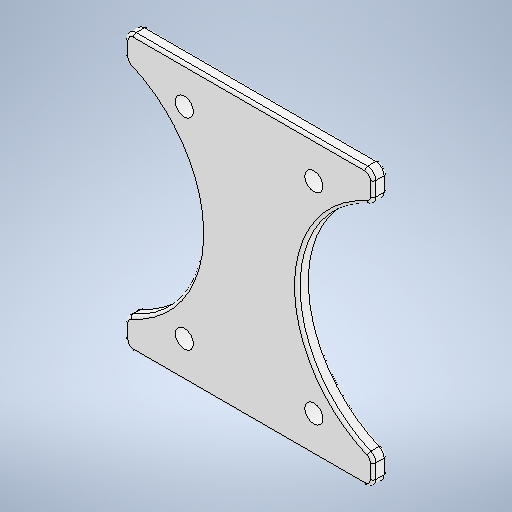
# Autodesk Inventor part: motor_clamp1
Saved by Autodesk Inventor 2025.3 (Build 293356030, 356C)
## iProperties
Created: 2025-11-17
Part Number: motor_clamp1
Material: PLA filament
Document SubType Name: Modeling
Designer: MSI
Mass: 47.447 g
Surface Area: 145.046 cm^2
Volume: 39.5392 cm^3
Density: 1.2 g/cm^3
Appearance: 일반
Author: MSI
Autodesk Inventor part; units mm, degrees
ref_plane "YZ Plane" through (0, 0, 0) normal (1, 0, 0) x (0, 1, 0)
ref_plane "XZ Plane" through (0, 0, 0) normal (0, 1, 0) x (-1, 0, 0)
ref_plane "XY Plane" through (0, 0, 0) normal (0, 0, 1) x (1, 0, 0)
sketch "스케치1" plane through (0, 0, 0) normal (0, 0, 1) x (1, 0, 0)
  line L0 (-45, 50) -> (45, 50)
  line L1 (45, 50) -> (45, -50)
  line L2 (45, -50) -> (-45, -50)
  line L3 (-45, -50) -> (-45, 50)
  line L4 (-45, 50) -> (45, -50) construction
  line L5 (45, 50) -> (-45, -50) construction
  point P0 (0, 0)
  dimension "d0" = 90
  dimension "d1" = 100
  constraints: 12 end point, 2 midpoint, 2 parallel, 1 horizontal, 1 perpendicular
  measures "d0" distance of L1.end L2.end
  measures "d1" distance of L0.end L1.end
extrude "돌출1" add sketch "스케치1" along normal mid plane 5
sketch "스케치2" plane through (0, 0, 2.5) normal (0, 0, 1) x (1, 0, 0)
  circle A0 centre (-60, 0) radius 42.5
  circle A1 centre (60, 0) radius 42.5
  point P0 (0, 0)
  dimension "d4" = 85
  dimension "d5" = 85
  dimension "d6" = 120
  dimension "d7" = 60
  constraints: 2 centre point, 2 horizontal alignment
  measures "d4" diameter of A0
  measures "d5" diameter of A1
  measures "d6" distance of A1.centre A0.centre
  measures "d7" distance of point (0, 0) A0.centre
extrude "돌출2" cut sketch "스케치2" against normal through all
sketch "스케치3" plane through (0, 0, 2.5) normal (0, 0, 1) x (1, 0, 0)
  line L0 (-23.5, 36.5) -> (23.5, 36.5) construction
  line L1 (23.5, 36.5) -> (23.5, -36.5) construction
  line L2 (23.5, -36.5) -> (-23.5, -36.5) construction
  line L3 (-23.5, -36.5) -> (-23.5, 36.5) construction
  line L4 (-23.5, 36.5) -> (23.5, -36.5) construction
  line L5 (23.5, 36.5) -> (-23.5, -36.5) construction
  point P0 (0, 0)
  dimension "d11" = 73
  dimension "d12" = 47
  constraints: 12 end point, 4 coincident, 2 midpoint, 2 parallel, 1 horizontal, 1 perpendicular
  measures "d11" distance of L0.end L1.end
  measures "d12" distance of L1.end L2.end
hole "구멍1" at (-23.5, 36.5, 2.5) at (23.5, 36.5, 2.5) at (23.5, -36.5, 2.5) at (-23.5, -36.5, 2.5) direction (0, 0, -1) diameter 6.6 end through all clearance for "Socket Head Cap Screw ISO 4762" size "M6" standard "ISO"
fillet "모깎기1" radius 3 8 edges at (45, -50, 0) (45, 50, 0) (45, 39.7649, 0) (-45, -50, 0) (45, -39.7649, 0) (-45, -39.7649, 0) (-45, 39.7649, 0) (-45, 50, 0)
fillet "모깎기2" radius 1 32 edges at (-44.1213, 49.1213, 2.5) (-45, 44.3941, 2.5) (-44.506, 40.139, 2.5) (-17.5, 0, 2.5) (-44.506, -40.139, 2.5) (-45, -44.3941, 2.5) (-44.1213, -49.1213, 2.5) (0, -50, 2.5) (44.1213, -49.1213, 2.5) (45, -44.3941, 2.5) (44.506, -40.139, 2.5) (17.5, 0, 2.5) (44.506, 40.139, 2.5) (45, 44.3941, 2.5) (44.1213, 49.1213, 2.5) (0, 50, 2.5) (-44.506, 40.139, -2.5) (-45, 44.3941, -2.5) (-44.1213, 49.1213, -2.5) (0, 50, -2.5) (44.1213, 49.1213, -2.5) (45, 44.3941, -2.5) (44.506, 40.139, -2.5) (17.5, 0, -2.5) (44.506, -40.139, -2.5) (45, -44.3941, -2.5) (44.1213, -49.1213, -2.5) (0, -50, -2.5) (-44.1213, -49.1213, -2.5) (-45, -44.3941, -2.5) (-44.506, -40.139, -2.5) (-17.5, 0, -2.5)
equation "\"d5\" = d4"
equation "\"d7\" = 0.5 * d6"
